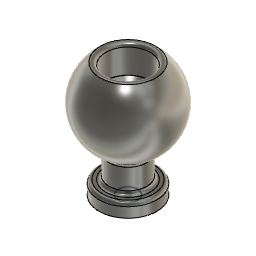
domekit_gheleguen_ball-joint_v2 (Autodesk Fusion 360 design; units mm, degrees)
Autodesk Fusion 360 part; units mm, degrees
sphere "SpherePrimitive1" add diameter 19.99 placed x (1, 0, 0) y (0, 0, -1) z (0, 1, 0) at (0, 0, 0)
sketch "Esquisse3" plane through (0, 0, 0) normal (0, 0, 1) x (1, 0, 0)
  circle A0 centre (0, 0) radius 4.25
  dimension "d3" = 8.5
  constraint coincident A0.centre origin
  measures "d3" diameter of A0
extrude "Extrusion1" add sketch "Esquisse3" against normal blind 18
sketch "Esquisse4" plane through (0, 0, -18) normal (0, 0, -1) x (1, 0, 0)
  circle A0 centre (0, 0) radius 4.25
  circle A1 centre (0, 0) radius 2.15
  dimension "d6" = 4.3
  constraint concentric A0 A1
  measures "d6" diameter of A1
extrude "Extrusion2" cut sketch "Esquisse4" against normal blind 30 contours A1
sketch "Esquisse5" plane through (0, 0, 0) normal (0, 0, 1) x (1, 0, 0)
  circle A0 through (5, 0, 9.761) (-2.5, 4.3301, 9.761) (-2.5, -4.3301, 9.761)
  circle A1 through (2.15, 0, 9.761) (-1.075, 1.862, 9.761) (-1.075, -1.862, 9.761)
  dimension "d12" = 10
extrude "Extrusion3" cut sketch "Esquisse5" against normal blind 8 contours A0 in plane through (0, 0, 9.761) normal (0, 0, 1)
chamfer "Chanfrein2" distance 2.8 angle 45 1 edges at (-2.0045, -0.7775, 1.761)
fillet "Congé1" radius 0.75 1 edges at (-4.6616, 1.8081, 8.6545)
chamfer "Chanfrein3" distance 0.25 angle 45 1 edges at (-3.9624, 1.5369, -18)
fillet "Congé2" radius 1 1 edges at (-3.9624, -1.5369, -9.0464)
sketch "Esquisse6" plane through (0, 0, -18) normal (0, 0, -1) x (1, 0, 0)
  circle A0 centre (0, 0) radius 2.15
  circle A1 centre (0, 0) radius 4
  circle A2 centre (0, 0) radius 6.5
  dimension "d21" = 13
  constraint coincident A0.centre A1.centre
  measures "d21" diameter of A2
extrude "Extrusion4" add sketch "Esquisse6" against normal blind 3 contours A2
fillet "Congé3" radius 0.75 1 edges at (-6.0601, -2.3505, -15)
fillet "Congé4" radius 0.75 1 edges at (-3.9624, -1.5369, -15)
